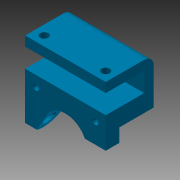
# Autodesk Inventor part: Part1
Saved by Autodesk Inventor 2015 (Build 190159000, 159)
## iProperties
Created: 2015-07-07
Part Number: Part1
Material: ABS Plastic
Document SubType Name: Modeling
Designer: eefred
Density: 1.06 g/cm^3
Appearance: Sky Blue Medium
Author: eefred
Autodesk Inventor part; units mm, degrees
ref_plane "YZ Plane" through (0, 0, 0) normal (1, 0, 0) x (0, 1, 0)
ref_plane "XZ Plane" through (0, 0, 0) normal (0, 1, 0) x (-1, 0, 0)
ref_plane "XY Plane" through (0, 0, 0) normal (0, 0, 1) x (1, 0, 0)
sketch "Sketch1" plane through (0, 0, 0) normal (1, 0, 0) x (0, 1, 0)
  line L0 (0, 0) -> (0, -5)
  line L1 (0, -5) -> (20, -5)
  line L2 (20, -5) -> (20, -15)
  line L3 (20, -15) -> (0, -15)
  line L4 (0, -15) -> (0, -39.4721)
  line L5 (25, 0) -> (25, -24)
  line L6 (25, -24) -> (7, -24)
  line L7 (7, -24) -> (7, -29.8038)
  line L8 (25, 0) -> (0, 0)
  circle A0 centre (4, -35) radius 3
  arc A1 (0, -39.4721) -> (7, -29.8038) centre (4, -35) ccw
  dimension "d0" = 5
  dimension "d1" = 20
  dimension "d2" = 10
  dimension "d5" = 5
  dimension "d6" = 7
  dimension "d7" = 6
  dimension "d8" = 20
  dimension "d9" = 4
  dimension "d10" = 6
  dimension "d45" = 9
  constraints: 18 end point, 3 perpendicular, 2 centre point, 2 horizontal, 2 point on circle, 2 point on line, 2 vertical, 1 coincident, 1 parallel
  measures "d0" distance of L0.start L0.end
  measures "d1" distance of L0.end L1.end
  measures "d2" distance of L1.end L2.end
  measures "d5" distance between parallel lines of L5 L2
  measures "d6" distance between parallel lines of L4 L7
  measures "d7" diameter of A0
  measures "d8" distance from line of L3 A0.centre
  measures "d9" distance from line of L4 A0.centre
  measures "d10" radius of A1
  measures "d45" distance between parallel lines of L6 L3
extrude "Extrusion1" add sketch "Sketch1" along normal blind 42
fillet "Fillet1" radius 5 1 edges at (21, 25, 0)
sketch "Sketch2" plane through (0, 7, -24) normal (0, 1, 0) x (1, 0, 0)
  arc A0 (10.8664, 7) -> (31.1336, 7) centre (21, 12) ccw
  line L0 (0, 0) -> (42, 0) projected
  line L1 (10.8664, 7) -> (3.3664, 19.9904)
  line L2 (10.8664, 7) -> (25.8664, 7) construction
  line L3 (31.1336, 7) -> (38.6336, 19.9904)
  line L4 (31.1336, 7) -> (46.1336, 7) construction
  line L5 (38.6336, 19.9904) -> (3.3664, 19.9904)
  line L6 (0, 0) -> (42, 0) projected
  point P0 (0, -24)
  point P1 (21, 0)
  dimension "d14" = 11.3
  dimension "d15" = 12
  dimension "d16" = 7
  dimension "d17" = 15
  dimension "d18" = 120
  dimension "d19" = 15
  dimension "d20" = 60
  constraints: 10 end point, 2 equal length, 2 horizontal, 2 point on circle, 1 centre point, 1 horizontal alignment, 1 midpoint, 1 vertical alignment
  measures "d14" radius of A0
  measures "d15" distance from line of A0.centre L0
  measures "d16" distance from line of L0 L1.start
  measures "d17" distance of L1.start L1.end
  measures "d18" angle of L2 L1
  measures "d19" distance of L3.start L3.end
  measures "d20" angle of L4 L3
extrude "Extrusion2" cut sketch "Sketch2" along normal through all both and the other way through all
sketch "Sketch3" plane through (42, 0, 0) normal (1, 0, 0) x (0, 0, -1)
  line L0 (29, 7) -> (31, 7)
  line L1 (31, 7) -> (31, 0)
  line L2 (31, 0) -> (43, 0)
  line L3 (43, 0) -> (43, 12)
  line L4 (43, 12) -> (29, 12)
  line L5 (29, 12) -> (29, 7)
  line L6 (15, 20) -> (15, 0) projected
  point P0 (0, 0)
  dimension "d23" = 7
  dimension "d24" = 16
  dimension "d25" = 2
  dimension "d26" = 12
  dimension "d27" = 14
  constraints: 12 end point, 5 perpendicular, 1 horizontal, 1 horizontal alignment
  measures "d23" distance between parallel lines of L2 L0
  measures "d24" distance between parallel lines of L6 L1
  measures "d25" distance of L0.start L0.end
  measures "d26" distance of L2.end L3.end
  measures "d27" distance of L3.end L4.end
extrude "Extrusion3" cut sketch "Sketch3" against normal up to surface
sketch "Sketch4" plane through (0, 25, -24) normal (0, 1, 0) x (1, 0, 0)
  circle A0 centre (5.5, -3.5) radius 1.6
  circle A1 centre (36.5, -3.5) radius 1.6
  line L0 (0, 0) -> (0, -19) projected
  line L1 (42, 0) -> (42, -19) projected
  line L2 (0, 0) -> (42, 0) projected
  point P0 (0, -24)
  dimension "d30" = 3.2
  dimension "d31" = 5.5
  dimension "d32" = 5.5
  dimension "d33" = 3.5
  dimension "d34" = 3.5
  constraints: 2 centre point, 1 equal radius
  measures "d30" diameter of A0
  measures "d31" distance from line of L0 A0.centre
  measures "d32" distance from line of L1 A1.centre
  measures "d33" distance from line of A1.centre L2
  measures "d34" distance from line of A0.centre L2
extrude "Extrusion4" cut sketch "Sketch4" against normal through all
sketch "Sketch5" plane through (0, 0, 0) normal (0, 0, 1) x (1, 0, 0)
  circle A0 centre (5, 5) radius 2.1
  circle A1 centre (37, 5) radius 2.1
  line L0 (0, 0) -> (42, 0) projected
  line L1 (0, 20) -> (0, 0) projected
  line L2 (42, 20) -> (42, 0) projected
  dimension "d37" = 4.2
  dimension "d38" = 5
  dimension "d39" = 5
  dimension "d40" = 5
  constraints: 2 centre point, 1 equal radius, 1 horizontal alignment
  measures "d37" diameter of A0
  measures "d38" distance from line of A0.centre L0
  measures "d39" distance from line of L1 A0.centre
  measures "d40" distance from line of L2 A1.centre
extrude "Extrusion5" cut sketch "Sketch5" against normal up to next
sketch "Sketch6" plane through (0, 25, -24) normal (0, 1, 0) x (1, 0, 0)
  spline S0 degree 2 poles (24.4322, -4.6341) (24.4322, -4.7612) (24.4049, -5.0608) knots 0 0 0 1 1 1
  spline S1 degree 2 poles (24.4049, -5.0608) (24.3777, -5.3696) (24.3777, -5.5149) knots 0 0 0 1 1 1
  spline S2 degree 2 poles (24.3777, -5.5149) (24.3777, -6.9405) (24.8045, -8.2754) knots 0 0 0 1 1 1
  spline S3 degree 2 poles (24.8045, -8.2754) (24.977, -8.8293) (24.977, -9.0654) knots 0 0 0 1 1 1
  spline S4 degree 2 poles (24.977, -9.0654) (24.977, -9.3832) (24.4776, -9.7374) (24.2506, -9.7374) knots 0 0 0 1 2 2 2
  spline S5 degree 2 poles (24.2506, -9.7374) (24.1507, -9.7374) (23.7693, -9.6465) knots 0 0 0 1 1 1
  spline S6 degree 2 poles (23.7693, -9.6465) (23.288, -9.5285) (22.6796, -9.4559) knots 0 0 0 1 1 1
  line L0 (22.6796, -9.4559) -> (18.3573, -8.9837)
  spline S7 degree 2 poles (18.3573, -8.9837) (17.7398, -8.9292) (17.3766, -8.8384) (17.086, -8.4752) (17.086, -8.1573) knots 0 0 0 1 2 3 3 3
  spline S8 degree 2 poles (17.086, -8.1573) (17.086, -7.9122) (17.4583, -7.5308) (17.6762, -7.5308) knots 0 0 0 1 2 2 2
  spline S9 degree 2 poles (17.6762, -7.5308) (17.876, -7.5308) (18.3845, -7.6307) knots 0 0 0 1 1 1
  spline S10 degree 2 poles (18.3845, -7.6307) (19.12, -7.7669) (23.2608, -8.2572) (23.3879, -8.2572) knots 0 0 0 1 2 2 2
  spline S11 degree 2 poles (23.3879, -8.2572) (23.5332, -8.2572) (23.5332, -8.2027) knots 0 0 0 1 1 1
  spline S12 degree 2 poles (23.5332, -8.2027) (23.5332, -8.003) (23.397, -7.1131) knots 0 0 0 1 1 1
  spline S13 degree 2 poles (23.397, -7.1131) (23.3243, -6.6954) (23.3062, -6.2686) knots 0 0 0 1 1 1
  spline S14 degree 2 poles (23.3062, -6.2686) (23.2517, -5.0518) (23.1246, -4.5614) knots 0 0 0 1 1 1
  spline S15 degree 2 poles (23.1246, -4.5614) (23.0882, -4.407) (23.0882, -4.3344) knots 0 0 0 1 1 1
  spline S16 degree 2 poles (23.0882, -4.3344) (23.0882, -4.0438) (23.4333, -3.7169) (23.6694, -3.7169) knots 0 0 0 1 2 2 2
  spline S17 degree 2 poles (23.6694, -3.7169) (24.0145, -3.7169) (24.4322, -4.2799) (24.4322, -4.6341) knots 0 0 0 1 2 2 2
  point P0 (0, -24)
  point P1 (17.086, -10.4002)
  constraints: 1 other
extrude "Extrusion6" add sketch "Sketch6" along normal blind 0.6
equation "\"d32\" = d31"
equation "\"d40\" = d39"
body "Solid1"
